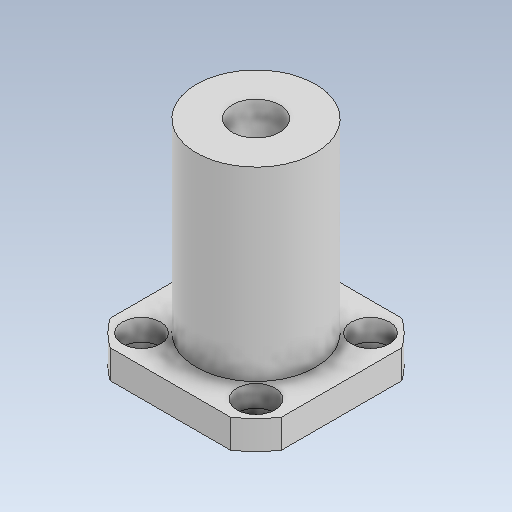
# Autodesk Inventor part: Peça28
Saved by Autodesk Inventor 2021 (Build 250183000, 183)
## iProperties
Category: 41
Created: 2021-07-21
Part Number: Peça28
Material: Genérico
Document SubType Name: Modeling
Designer: Giovanni
Density: 1 g/cm^3
Appearance: Padrão
User Status: 1:1
Author: Giovanni
Keywords: 30
Autodesk Inventor part; units mm, degrees
ref_plane "YZ Plane" through (0, 0, 0) normal (1, 0, 0) x (0, 1, 0)
ref_plane "XZ Plane" through (0, 0, 0) normal (0, 1, 0) x (-1, 0, 0)
ref_plane "XY Plane" through (0, 0, 0) normal (0, 0, 1) x (1, 0, 0)
sketch "Esboço1" plane through (0, 0, 0) normal (0, 0, 1) x (1, 0, 0)
  line L0 (0, 0) -> (0, 50)
  line L1 (-8.5, 0) -> (-8.5, 37)
  line L2 (-8.5, 37) -> (-5, 37)
  line L3 (-5, 37) -> (-5, 50)
  line L4 (-8.5, 0) -> (-12.5, 0)
  line L5 (-12.5, 0) -> (-12.5, 5)
  line L6 (-12.5, 5) -> (-22, 5)
  line L7 (-22, 5) -> (-22, 11)
  line L8 (-22, 11) -> (-12.5, 11)
  line L9 (-12.5, 11) -> (-12.5, 50)
  line L10 (-12.5, 50) -> (-5, 50)
  dimension "d0" = 50
  dimension "d1" = 17
  dimension "d2" = 10
  dimension "d3" = 13
  dimension "d4" = 25
  dimension "d5" = 44
  dimension "d6" = 5
  dimension "d7" = 6
  constraints: 22 end point, 5 perpendicular, 2 horizontal alignment, 2 point on line, 2 vertical
  measures "d0" distance of L0.start L0.end
  measures "d1" diameter of L1 L0
  measures "d2" diameter of L3 L0
  measures "d3" distance from line of L3.end L2
  measures "d4" diameter of L4.end L0
  measures "d5" diameter of L7 L0
  measures "d6" vertical distance of L4.end L6.end
  measures "d7" distance of L6.end L7.end
revolve "Revolução1" add sketch "Esboço1" angle 360 about axis through (0, 0, 0) along (0, 1, 0)
sketch "Esboço2" plane through (0, 11, 0) normal (0, 1, 0) x (1, 0, 0)
  circle A0 centre (0, 0) radius 22 projected
  circle A1 centre (0, 0) radius 12.5 projected
  line L0 (-12.6491, 18) -> (12.6491, 18)
  arc A2 (12.6491, 18) -> (-12.6491, 18) centre (0, 0) ccw
  dimension "d9" = 18
  constraints: 4 point on circle, 2 end point, 1 centre point, 1 coincident, 1 concentric, 1 horizontal
  measures "d9" distance from line of A0.centre L0
extrude "Extrusão1" cut sketch "Esboço2" against normal up to next contours L0 A0 picked at (-0.8962, 19.2784)
pattern_circular "Padrão circular1" count 4 over 360 about axis through (0, -10, 0) along (0, 1, 0) of "Extrusão1"
sketch "Esboço3" plane through (-12.6491, 11, -18) normal (0, 1, 0) x (1, 0, 0)
  circle A0 centre (12.6491, -18) radius 12.5 projected
  line L0 (24.6699, -30.0208) -> (12.6491, -18)
  line L1 (12.6491, -18) -> (30.6491, -18)
  line L2 (30.6491, -5.3509) -> (30.6491, -30.6491) projected
  dimension "d15" = 45
  dimension "d16" = 17
  constraints: 4 end point, 1 midpoint
  measures "d15" angle of L0 L1
  measures "d16" distance of L0.start L0.end
hole "Furo1" at (12.0208, 11, 12.0208) direction (0, -1, 0) diameter 4.5 end through all counterbore diameter 8 counterbore depth 4.5 clearance for "Socket Head Cap Screw DIN EN ISO 4762" size "M4" standard "DIN"
pattern_circular "Padrão circular2" count 4 over 360 about axis through (0, -10, 0) along (0, 1, 0) of "Furo1"
